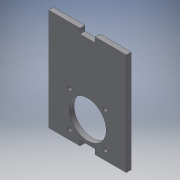
# Autodesk Inventor part: side_plate
Saved by Autodesk Inventor 2017 (Build 210142000, 142)
## iProperties
Created: 2017-06-15
Part Number: side_plate
Material: Generic
Document SubType Name: Modeling
Designer: millerid
Density: 1 g/cm^3
Appearance: Default
Author: millerid
Autodesk Inventor part; units mm, degrees
ref_plane "YZ Plane" through (0, 0, 0) normal (1, 0, 0) x (0, 1, 0)
ref_plane "XZ Plane" through (0, 0, 0) normal (0, 1, 0) x (-1, 0, 0)
ref_plane "XY Plane" through (0, 0, 0) normal (0, 0, 1) x (1, 0, 0)
sketch "Sketch1" plane through (0, 0, 0) normal (0, 0, 1) x (1, 0, 0)
  line L0 (50.2032, 0) -> (50.2032, 60)
  line L1 (0, 60) -> (0, 0)
  line L2 (20.2032, 0.2766) -> (20.2032, -3)
  line L3 (20.2032, -3) -> (0, -3)
  line L4 (0, -3) -> (0, 0)
  line L5 (30, 0.2766) -> (30, -3)
  line L6 (30, -3) -> (50.2032, -3)
  line L7 (50.2032, -3) -> (50.2032, 0)
  line L8 (20.2032, 0.2766) -> (30, 0.2766)
  line L9 (20.2032, 59.7234) -> (20.2032, 63)
  line L10 (20.2032, 63) -> (0, 63)
  line L11 (0, 63) -> (0, 60)
  line L12 (30, 59.7234) -> (30, 63)
  line L13 (30, 63) -> (50.2032, 63)
  line L14 (50.2032, 63) -> (50.2032, 60)
  line L15 (30, 59.7234) -> (20.2032, 59.7234)
  circle A0 centre (25.2032, 14.2766) radius 12
  circle A1 centre (13.6016, 2.8766) radius 1.25
  circle A2 centre (36.6016, 2.8766) radius 1.25
  circle A3 centre (13.6016, 25.8766) radius 1.25
  circle A4 centre (36.5, 25.6) radius 1.25
  point P0 (25.1016, 0.2766)
  dimension "d1" = 60
  dimension "d2" = 20.2032
  dimension "d3" = 3.2766
  dimension "d4" = 20.2032
  dimension "d5" = 20.2032
  dimension "d6" = 3.2766
  dimension "d7" = 20.2032
  dimension "d8" = 24
  dimension "d9" = 14
  dimension "d10" = 25
  dimension "d11" = 2.5
  dimension "d12" = 2.6
  dimension "d13" = 11.5
  dimension "d14" = 2.5
  dimension "d15" = 11.5
  dimension "d16" = 2.5
  dimension "d17" = 23
  dimension "d18" = 2.5
  dimension "d21" = 50.2032
  constraints: 32 end point, 5 centre point, 5 parallel, 2 horizontal, 2 point on line, 1 midpoint
  measures "d1" distance of L0.end L0.start
  measures "d2" distance of L2.end L3.end
  measures "d3" distance of L2.start L2.end
  measures "d4" distance of L6.end L5.end
  measures "d5" distance of L10.end L9.end
  measures "d6" distance of L9.end L9.start
  measures "d7" distance of L12.end L13.end
  measures "d8" diameter of A0
  measures "d9" distance from line of A0.centre L8
  measures "d10" distance from line of L0 A0.centre
  measures "d11" diameter of A1
  measures "d12" distance from line of L8 A1.centre
  measures "d13" horizontal distance of A1.centre point (25.102, 0.277)
  measures "d14" diameter of A2
  measures "d15" horizontal distance of A2.centre point (25.102, 0.277)
  measures "d16" diameter of A3
  measures "d17" distance of A1.centre A3.centre
  measures "d18" diameter of A4
  measures "d21" distance between parallel lines of L0 L1
extrude "Extrusion1" add sketch "Sketch1" along normal blind 3.175
equation "\"d4\" = d2"
equation "\"d5\" = d2"
equation "\"d6\" = d3"
equation "\"d7\" = d2"
equation "\"d15\" = d13"
body "Solid1"
